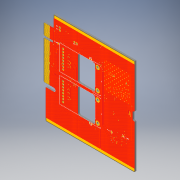
# Autodesk Inventor part: CardStandard
Saved by Autodesk Inventor 2018 (Build 220112000, 112)
## iProperties
Created: 2018-01-15
Part Number: CardStandard
Material: Epoxy Resin
Document SubType Name: Modeling
Designer: Bradley
Density: 1.14 g/cm^3
Appearance: Smooth - Medium Gray
Mass: 15.4834 g
Surface Area: 175.95 cm^2
Volume: 13.582 cm^3
Author: Bradley
Revision Number: 3.1
Autodesk Inventor part; units mm, degrees
ref_plane "YZ Plane" through (0, 0, 0) normal (1, 0, 0) x (0, 1, 0)
ref_plane "XZ Plane" through (0, 0, 0) normal (0, 1, 0) x (-1, 0, 0)
ref_plane "XY Plane" through (0, 0, 0) normal (0, 0, 1) x (1, 0, 0)
sketch "Sketch1" plane through (0, 0, 0) normal (0, 0, 1) x (1, 0, 0)
  line L0 (0, 36.15) -> (10, 36.15)
  line L1 (10, 36.15) -> (10, 47.9)
  line L2 (10, 47.9) -> (90.4, 47.9)
  line L3 (90.4, 47.9) -> (90.4, -47.9)
  line L4 (90.4, -47.9) -> (2, -47.9)
  line L5 (10, -15.15) -> (0, -15.15)
  line L6 (-5.5, 48) -> (90.5, 48) construction
  line L7 (90.5, 48) -> (90.5, -48) construction
  line L8 (90.5, -48) -> (-5.5, -48) construction
  line L9 (-5.5, -48) -> (-5.5, 48) construction
  line L10 (-5.4, 47.9) -> (-3.4, 47.9) construction
  line L11 (-3.4, 47.9) -> (-3.4, -47.9) construction
  line L12 (-3.4, -47.9) -> (-5.4, -47.9) construction
  line L13 (-5.4, -47.9) -> (-5.4, 47.9) construction
  line L14 (-3.4, 38.5) -> (7.85, 38.5) construction
  line L15 (7.85, 38.5) -> (7.85, -17.5) construction
  line L16 (7.85, -17.5) -> (-3.4, -17.5) construction
  line L17 (-3.4, -17.5) -> (-3.4, 38.5) construction
  line L18 (2, -47.9) -> (2, -18.65)
  line L19 (2, -18.65) -> (10, -18.65)
  arc A0 (10, -18.65) -> (10, -15.15) centre (10, -16.9) ccw
  line L20 (0, 24) -> (90.5, 24) construction
  circle A1 centre (-2.5, 47.1) radius 0.9 construction
  circle A2 centre (-0.7, 47.1) radius 0.9 construction
  circle A3 centre (1.1, 47.1) radius 0.9 construction
  circle A4 centre (2.9, 47.1) radius 0.9 construction
  circle A5 centre (4.7, 47.1) radius 0.9 construction
  circle A6 centre (6.5, 47.1) radius 0.9 construction
  circle A7 centre (8.3, 47.1) radius 0.9 construction
  circle A8 centre (-2.5, 45.3) radius 0.9 construction
  circle A9 centre (-0.7, 45.3) radius 0.9 construction
  circle A10 centre (1.1, 45.3) radius 0.9 construction
  circle A11 centre (2.9, 45.3) radius 0.9 construction
  circle A12 centre (4.7, 45.3) radius 0.9 construction
  circle A13 centre (6.5, 45.3) radius 0.9 construction
  circle A14 centre (8.3, 45.3) radius 0.9 construction
  circle A15 centre (-2.5, 43.5) radius 0.9 construction
  circle A16 centre (-0.7, 43.5) radius 0.9 construction
  circle A17 centre (1.1, 43.5) radius 0.9 construction
  circle A18 centre (2.9, 43.5) radius 0.9 construction
  circle A19 centre (4.7, 43.5) radius 0.9 construction
  circle A20 centre (6.5, 43.5) radius 0.9 construction
  circle A21 centre (8.3, 43.5) radius 0.9 construction
  circle A22 centre (-2.5, 41.7) radius 0.9 construction
  circle A23 centre (-0.7, 41.7) radius 0.9 construction
  circle A24 centre (1.1, 41.7) radius 0.9 construction
  circle A25 centre (2.9, 41.7) radius 0.9 construction
  circle A26 centre (4.7, 41.7) radius 0.9 construction
  circle A27 centre (6.5, 41.7) radius 0.9 construction
  circle A28 centre (8.3, 41.7) radius 0.9 construction
  circle A29 centre (-2.5, 39.9) radius 0.9 construction
  circle A30 centre (-0.7, 39.9) radius 0.9 construction
  circle A31 centre (1.1, 39.9) radius 0.9 construction
  circle A32 centre (2.9, 39.9) radius 0.9 construction
  circle A33 centre (4.7, 39.9) radius 0.9 construction
  circle A34 centre (6.5, 39.9) radius 0.9 construction
  circle A35 centre (8.3, 39.9) radius 0.9 construction
  line L21 (0, 36.15) -> (0, 24.95)
  line L22 (0, 24.95) -> (8.4, 24.95)
  arc A36 (8.4, 23.05) -> (8.4, 24.95) centre (8.4, 24) ccw
  line L23 (8.4, 23.05) -> (0, 23.05)
  line L24 (0, 23.05) -> (0, -15.15)
  point P0 (0, 0)
  point P1 (-5.5, 0)
  point P2 (90.4, 0)
  point P3 (90.5, 0)
  dimension "d0" = 51.3
  dimension "d1" = 95.8
  dimension "d3" = 10
  dimension "d20" = 96
  dimension "d21" = 96
  dimension "d22" = 0.1
  dimension "d23" = 0.1
  dimension "d24" = 2
  dimension "d25" = 0.1
  dimension "d28" = 11.25
  dimension "d29" = 56
  dimension "d31" = 9.5
  dimension "d32" = 30.5
  dimension "d34" = 3.5
  dimension "d35" = 12.15
  dimension "d36" = 39.15
  dimension "d37" = 14.5
  dimension "d38" = 1.15
  dimension "d39" = 1.8
  dimension "d42" = 1.8
  dimension "d45" = 1.8
  dimension "d48" = 2
  dimension "d49" = 3.4
  dimension "d50" = 1.9
  dimension "d51" = 8.4
  dimension "d52" = 24
  constraints: 50 end point, 37 centre point, 11 perpendicular, 7 parallel, 6 point on line, 6 tangent, 5 horizontal, 4 point on circle, 3 midpoint, 3 vertical, 2 collinear, 2 horizontal alignment, 68 other
  measures "d0" distance of L5.end L0.start
  measures "d1" distance of L2.end L3.end
  measures "d3" distance of L0.start L0.end
  measures "d20" distance of L6.start L6.end
  measures "d21" distance of L8.end L6.start
  measures "d22" distance between parallel lines of L2 L6
  measures "d23" distance between parallel lines of L7 L3
  measures "d24" distance between parallel lines of L13 L11
  measures "d25" distance between parallel lines of L13 L9
  measures "d28" distance of L15.end L16.end
  measures "d29" distance of L14.end L15.end
  measures "d31" distance between parallel lines of L14 L6
  measures "d32" distance between parallel lines of L8 L16
  measures "d34" distance between parallel lines of L5 L19
  measures "d35" distance between parallel lines of L20 L0
  measures "d36" distance between parallel lines of L5 L20
  measures "d37" distance between parallel lines of L20 L14
  measures "d38" distance between parallel lines of L19 L16
  measures "d39" diameter of A1
  measures "d42" distance of A1.centre A2.centre
  measures "d45" distance of A1.centre A8.centre
  measures "d48" distance between parallel lines of L18 L24
  measures "d49" distance between parallel lines of L24 L11
  measures "d50" distance between parallel lines of L23 L22
  measures "d51" distance of L21.end L22.end
  measures "d52" distance from line of point (0, 0) L20
extrude "Extrusion1" add sketch "Sketch1" along normal mid plane 1.6
chamfer "Chamfer1" distance 0.5 angle 45 4 edges at (0, 36.15, 0) (0, 24.95, 0) (0, 23.05, 0) (0, -15.15, 0)
fillet "Fillet1" radius 0.5 6 edges at (10, 36.15, 0) (10, 47.9, 0) (90.4, 47.9, 0) (90.4, -47.9, 0) (2, -47.9, 0) (2, -18.65, 0)
sketch "Sketch16" plane through (0, 0, 0.8) normal (0, 0, 1) x (1, 0, 0)
  arc A0 (2.5, -18.65) -> (2, -19.15) centre (2.5, -19.15) ccw projected
  line L0 (2, -19.15) -> (2, -47.4) projected
  arc A1 (2, -47.4) -> (2.5, -47.9) centre (2.5, -47.4) ccw projected
  line L1 (2.5, -47.9) -> (89.9, -47.9) projected
  arc A2 (89.9, -47.9) -> (90.4, -47.4) centre (89.9, -47.4) ccw projected
  line L2 (90.4, -47.4) -> (90.4, 47.4) projected
  arc A3 (90.4, 47.4) -> (89.9, 47.9) centre (89.9, 47.4) ccw projected
  line L3 (89.9, 47.9) -> (10.5, 47.9) projected
  arc A4 (10.5, 47.9) -> (10, 47.4) centre (10.5, 47.4) ccw projected
  line L4 (10, 47.4) -> (10, 36.65) projected
  arc A5 (9.5, 36.15) -> (10, 36.65) centre (9.5, 36.65) ccw projected
  line L5 (9.5, 36.15) -> (0.5, 36.15) projected
  line L6 (0, 35.65) -> (0.5, 36.15) projected
  line L7 (0, 35.65) -> (0, 25.45) projected
  line L8 (0.5, 24.95) -> (0, 25.45) projected
  line L9 (0.5, 24.95) -> (8.4, 24.95) projected
  arc A6 (8.4, 23.05) -> (8.4, 24.95) centre (8.4, 24) ccw projected
  line L10 (8.4, 23.05) -> (0.5, 23.05) projected
  line L11 (0, 22.55) -> (0.5, 23.05) projected
  line L12 (0, 22.55) -> (0, -14.65) projected
  line L13 (0.5, -15.15) -> (0, -14.65) projected
  line L14 (0.5, -15.15) -> (10, -15.15) projected
  arc A7 (10, -18.65) -> (10, -15.15) centre (10, -16.9) ccw projected
  line L15 (10, -18.65) -> (2.5, -18.65) projected
  line L16 (36.05, 26.5) -> (49.05, 26.5)
  line L17 (51.05, 24.5) -> (51.05, 3.5)
  line L18 (49.05, 1.5) -> (36.05, 1.5)
  line L19 (34.05, 3.5) -> (34.05, 24.5)
  line L20 (36.05, -1.5) -> (49.05, -1.5)
  line L21 (51.05, -3.5) -> (51.05, -24.5)
  line L22 (49.05, -26.5) -> (36.05, -26.5)
  line L23 (34.05, -24.5) -> (34.05, -3.5)
  line L24 (88.4, 3) -> (88.4, -3)
  arc A8 (88.4, -3) -> (89.4, -4) centre (89.4, -3) ccw
  arc A9 (90.4, -5) -> (89.4, -4) centre (89.4, -5) ccw
  arc A10 (89.4, 4) -> (88.4, 3) centre (89.4, 3) ccw
  line L25 (90.4, -47.4) -> (90.4, 47.4) projected
  arc A11 (89.4, 4) -> (90.4, 5) centre (89.4, 5) ccw
  arc A12 (36.05, 26.5) -> (34.05, 24.5) centre (36.05, 24.5) ccw
  arc A13 (51.05, 24.5) -> (49.05, 26.5) centre (49.05, 24.5) ccw
  arc A14 (49.05, 1.5) -> (51.05, 3.5) centre (49.05, 3.5) ccw
  arc A15 (51.05, -3.5) -> (49.05, -1.5) centre (49.05, -3.5) ccw
  arc A16 (49.05, -26.5) -> (51.05, -24.5) centre (49.05, -24.5) ccw
  arc A17 (34.05, -24.5) -> (36.05, -26.5) centre (36.05, -24.5) ccw
  arc A18 (36.05, -1.5) -> (34.05, -3.5) centre (36.05, -3.5) ccw
  arc A19 (34.05, 3.5) -> (36.05, 1.5) centre (36.05, 3.5) ccw
  point P0 (0, 0)
  point P1 (34.05, -1.5)
  point P2 (51.05, -26.5)
  point P3 (88.4, 0)
  dimension "d145" = 6
  dimension "d146" = 1
  dimension "d147" = 3
  dimension "d148" = 1.5
  dimension "d149" = 34.05
  dimension "d150" = 51.05
  dimension "d151" = 26.5
  dimension "d152" = 2
  constraints: 24 point on circle, 22 tangent, 18 end point, 12 centre point, 10 equal radius, 8 point on line, 4 parallel, 2 horizontal, 2 perpendicular, 1 collinear, 1 horizontal alignment, 1 midpoint, 1 vertical, 1 vertical alignment
  measures "d145" distance of L24.start L24.end
  measures "d146" radius of A11
  measures "d147" distance between parallel lines of L20 L18
  measures "d148" distance from line of point (0, 0) L18
  measures "d149" distance between parallel lines of L19 L12
  measures "d150" distance between parallel lines of L12 L17
  measures "d151" distance from line of point (0, 0) L22
  measures "d152" radius of A12
extrude "Extrusion6" cut sketch "Sketch16" against normal through all contours A9 A8 L24 A10 A11 L2 | L16 A13 L17 A14 L18 A19 L19 A12 | L20 A15 L21 A16 L22 A17 L23 A18
sketch "Sketch19" plane through (0, 0, 0.8) normal (0, 0, 1) x (1, 0, 0)
  line L0 (0, 22.55) -> (0, -14.65) projected
  line L1 (90.4, 5) -> (90.4, 47.4) projected
  line L2 (0, 47.8927) -> (90.4, 47.8927) construction
  line L3 (90.4, 47.8927) -> (90.4, -47.8927) construction
  line L4 (90.4, -47.8927) -> (0, -47.8927) construction
  line L5 (0, -47.8927) -> (0, 47.8927) construction
  point P0 (0, 0)
  constraints: 2 collinear, 1 midpoint, 2 other
decal "Decal4"
sketch "Sketch20" plane through (0, 0, -0.8) normal (0, 0, -1) x (-1, 0, 0)
  line L0 (-90.4, 47.4) -> (-90.4, 5) projected
  line L1 (0, -14.65) -> (0, 22.55) projected
  line L2 (-90.4, 47.8927) -> (0, 47.8927) construction
  line L3 (0, 47.8927) -> (0, -47.8927) construction
  line L4 (0, -47.8927) -> (-90.4, -47.8927) construction
  line L5 (-90.4, -47.8927) -> (-90.4, 47.8927) construction
  point P0 (0, 0)
  constraints: 2 collinear, 1 midpoint, 2 other
decal "Decal5"
sketch "Sketch21" plane through (0, 0, 0.8) normal (0, 0, 1) x (1, 0, 0)
  point P0 (0, 0)
  point P1 (53.55, -24)
  point P2 (53.55, -4)
  point P3 (53.55, 24)
  point P4 (53.55, 4)
  constraints: 4 other
hole "Hole9" at (53.55, -24, 0.8) at (53.55, -4, 0.8) at (53.55, 24, 0.8) at (53.55, 4, 0.8) direction (0, 0, -1) diameter 2.2 end through all
sketch "Sketch22" plane through (0, 0, 0.8) normal (0, 0, 1) x (1, 0, 0)
  point P0 (0, 0)
  point P1 (19.25, -17.81)
  point P2 (32.9, 34.25)
  point P3 (19.25, -12.73)
  point P4 (19.25, -10.19)
  point P5 (19.25, -7.65)
  point P6 (19.25, -5.11)
  point P7 (19.25, -15.27)
  point P8 (19.25, 20.35)
  point P9 (19.25, -20.35)
  point P10 (19.25, -22.89)
  point P11 (19.25, 17.81)
  point P12 (19.25, 15.27)
  point P13 (19.25, 22.89)
  point P14 (19.25, 12.73)
  point P15 (19.25, 10.19)
  point P16 (19.25, 7.65)
  point P17 (19.25, 5.11)
  point P18 (30.5, 34.25)
  point P19 (16, 39.5)
  point P20 (16, 37.05)
  constraints: 20 other
hole "Hole10" at (19.25, -17.81, 0.8) at (32.9, 34.25, 0.8) at (19.25, -12.73, 0.8) at (19.25, -10.19, 0.8) at (19.25, -7.65, 0.8) at (19.25, -5.11, 0.8) at (19.25, -15.27, 0.8) at (19.25, 20.35, 0.8) at (19.25, -20.35, 0.8) at (19.25, -22.89, 0.8) at (19.25, 17.81, 0.8) at (19.25, 15.27, 0.8) at (19.25, 22.89, 0.8) at (19.25, 12.73, 0.8) at (19.25, 10.19, 0.8) at (19.25, 7.65, 0.8) at (19.25, 5.11, 0.8) at (30.5, 34.25, 0.8) at (16, 39.5, 0.8) at (16, 37.05, 0.8) direction (0, 0, -1) diameter 1 end through all
sketch "Sketch23" plane through (0, 0, 0.8) normal (0, 0, 1) x (1, 0, 0)
  point P0 (0, 0)
  point P1 (82, 24.5)
  point P2 (69.5, 24.5)
  constraints: 2 other
hole "Hole11" at (82, 24.5, 0.8) at (69.5, 24.5, 0.8) direction (0, 0, -1) diameter 0.6 end through all
sketch "Sketch24" plane through (0, 0, 0.8) normal (0, 0, 1) x (1, 0, 0)
  point P0 (0, 0)
  point P1 (52.419, -22.869)
  point P2 (51.95, -24)
  point P3 (52.419, -25.131)
  point P4 (55.15, -24)
  point P5 (53.55, -5.6)
  point P6 (54.681, -5.131)
  point P7 (55.15, -4)
  point P8 (54.681, -2.869)
  point P9 (53.55, -2.4)
  point P10 (52.419, -2.869)
  point P11 (54.681, -22.869)
  point P12 (53.55, 22.4)
  point P13 (54.681, 22.869)
  point P14 (55.15, 24)
  point P15 (54.681, 25.131)
  point P16 (53.55, 25.6)
  point P17 (52.419, 25.131)
  point P18 (51.95, -4)
  point P19 (52.419, 22.869)
  point P20 (53.55, 2.4)
  point P21 (54.681, 2.869)
  point P22 (55.15, 4)
  point P23 (54.681, 5.131)
  point P24 (53.55, 5.6)
  point P25 (51.95, 24)
  point P26 (51.95, 4)
  point P27 (52.419, 2.869)
  point P28 (52.419, -5.131)
  point P29 (53.55, -25.6)
  point P30 (54.681, -25.131)
  point P31 (53.55, -22.4)
  point P32 (52.419, 5.131)
  constraints: 32 other
hole "Hole12" at (52.419, -22.869, 0.8) at (51.95, -24, 0.8) at (52.419, -25.131, 0.8) at (55.15, -24, 0.8) at (53.55, -5.6, 0.8) at (54.681, -5.131, 0.8) at (55.15, -4, 0.8) at (54.681, -2.869, 0.8) at (53.55, -2.4, 0.8) at (52.419, -2.869, 0.8) at (54.681, -22.869, 0.8) at (53.55, 22.4, 0.8) at (54.681, 22.869, 0.8) at (55.15, 24, 0.8) at (54.681, 25.131, 0.8) at (53.55, 25.6, 0.8) at (52.419, 25.131, 0.8) at (51.95, -4, 0.8) at (52.419, 22.869, 0.8) at (53.55, 2.4, 0.8) at (54.681, 2.869, 0.8) at (55.15, 4, 0.8) at (54.681, 5.131, 0.8) at (53.55, 5.6, 0.8) at (51.95, 24, 0.8) at (51.95, 4, 0.8) at (52.419, 2.869, 0.8) at (52.419, -5.131, 0.8) at (53.55, -25.6, 0.8) at (54.681, -25.131, 0.8) at (53.55, -22.4, 0.8) at (52.419, 5.131, 0.8) direction (0, 0, -1) diameter 0.35 end through all
sketch "Sketch25" plane through (0, 0, 0.8) normal (0, 0, 1) x (1, 0, 0)
  point P0 (0, 0)
  point P1 (80.65, 14.55)
  point P2 (79.45, 14.55)
  point P3 (79.15, 12.8)
  point P4 (79.1, 11.55)
  point P5 (77.3, 14.15)
  point P6 (76.1, 14.15)
  point P7 (77.25, 12.15)
  point P8 (77.25, 10.95)
  point P9 (74.55, 13)
  point P10 (72.7, 14.55)
  point P11 (69.6, 14.35)
  point P12 (69.8, 13)
  point P13 (69.8, 11.1)
  point P14 (72.3, 11.4)
  point P15 (66.9, 23.8)
  point P16 (68.5, 23.8)
  point P17 (64.9, 24.9)
  point P18 (68.5, 25.1)
  point P19 (66.9, 25.1)
  point P20 (64.9, 23.6)
  point P21 (82.7, 23.6)
  point P22 (81.3, 23.6)
  point P23 (82, 25.6)
  point P24 (82.7, 19.4)
  point P25 (81.3, 18.8)
  point P26 (83.8, 16.4)
  point P27 (85, 17)
  point P28 (85.05, 14.2)
  point P29 (81.1, 16.2)
  point P30 (77.95, 16.35)
  point P31 (75.05, 16.35)
  point P32 (71.85, 15.55)
  point P33 (66.5, 13.7)
  point P34 (65.6, 12.3)
  point P35 (70.6, 24.5)
  point P36 (84.5, 32)
  point P37 (76.5, 32)
  point P38 (68.5, 32)
  point P39 (72.5, 32)
  point P40 (80.5, 32)
  point P41 (64.5, 32)
  point P42 (82.5, 30)
  point P43 (74.5, 30)
  point P44 (66.5, 30)
  point P45 (70.5, 30)
  point P46 (78.5, 30)
  point P47 (62.5, 30)
  point P48 (84.5, 28)
  point P49 (76.5, 28)
  point P50 (68.5, 28)
  point P51 (72.5, 28)
  point P52 (80.5, 28)
  point P53 (64.5, 28)
  point P54 (74.5, 26)
  point P55 (66.5, 26)
  point P56 (70.5, 26)
  point P57 (78.5, 26)
  point P58 (62.5, 26)
  point P59 (84.5, 24)
  point P60 (76.5, 24)
  point P61 (72.5, 24)
  point P62 (74.5, 22)
  point P63 (66.5, 22)
  point P64 (70.5, 22)
  point P65 (78.5, 22)
  point P66 (62.5, 22)
  point P67 (84.5, 20)
  point P68 (76.5, 20)
  point P69 (68.5, 20)
  point P70 (72.5, 20)
  point P71 (80.5, 20)
  point P72 (64.5, 20)
  point P73 (74.5, 18)
  point P74 (66.5, 18)
  point P75 (70.5, 18)
  point P76 (78.5, 18)
  point P77 (62.5, 18)
  point P78 (84.5, 8)
  point P79 (76.5, 8)
  point P80 (68.5, 8)
  point P81 (72.5, 8)
  point P82 (80.5, 8)
  point P83 (64.5, 8)
  point P84 (82.5, 10)
  point P85 (74.5, 10)
  point P86 (66.5, 10)
  point P87 (70.5, 10)
  point P88 (78.5, 10)
  point P89 (62.5, 10)
  point P90 (82.5, 34)
  point P91 (74.5, 34)
  point P92 (66.5, 34)
  point P93 (70.5, 34)
  point P94 (56.2, 27.1)
  point P95 (62.5, 34)
  point P96 (60.5, 32)
  point P97 (60.5, 28)
  point P98 (60.5, 24)
  point P99 (60.5, 20)
  point P100 (60.5, 16)
  point P101 (62.5, 14)
  point P102 (60.5, 12)
  point P103 (64.5, 12)
  point P104 (64.5, 16)
  point P105 (13.5, 24.2)
  point P106 (15.3, 2.5)
  point P107 (15.3, -4.8)
  point P108 (55.3, -27)
  point P109 (73.075, -22.125)
  point P110 (77.7, -26.1)
  point P111 (25, 9.9)
  point P112 (25, 12.8)
  point P113 (25, 15.9)
  point P114 (24.59, 18.9)
  point P115 (24.6, -9.1)
  point P116 (25, -18.1)
  point P117 (25, -15.1)
  point P118 (25, -12.1)
  point P119 (80.4, -20.2)
  point P120 (80.4, -17.9)
  point P121 (62.6, 1.8)
  point P122 (60.2, 3.5)
  point P123 (25.25, 1.4)
  point P124 (25.25, -1.4)
  point P125 (28.5, 1.4)
  point P126 (13.8, 20)
  point P127 (67.5, -26.2)
  point P128 (58.86, 23)
  point P129 (67, -31)
  point P130 (72.9, -30.3)
  point P131 (69.3, -28.5)
  point P132 (67, -28.5)
  point P133 (55.5, 29.3)
  point P134 (57.7, 27.5)
  point P135 (57.7, 25.6)
  point P136 (72.5, -32.1)
  point P137 (87.6, 7.7)
  point P138 (70.3, -30.7)
  point P139 (68.7, -33.25)
  point P140 (70.432, -27.94)
  point P141 (77.1, -30.9)
  point P142 (72.3, -26.4)
  point P143 (58.3, 24.9)
  point P144 (67, -32.3)
  point P145 (72.4, -30.9)
  point P146 (69.3, -29.8)
  point P147 (51.75, -29.75)
  point P148 (70.001, -7.599)
  point P149 (69.209, -8.391)
  point P150 (77.45, -23.85)
  point P151 (6, -2.5)
  point P152 (30.5, -2.4)
  point P153 (26.4, 14.45)
  point P154 (6, -3.5)
  point P155 (31.1, -3)
  point P156 (29.9, -3)
  point P157 (29.9, -1.8)
  point P158 (26.4, 13.6)
  point P159 (6, -4.5)
  point P160 (31.7, -3.6)
  point P161 (29.3, -3.6)
  point P162 (29.3, -1.2)
  point P163 (26.4, 11.45)
  point P164 (58, 30.4)
  point P165 (17.6, 8.9)
  point P166 (26.4, 10.1)
  point P167 (9.8, 5.2)
  point P168 (20.7, -1.4)
  point P169 (24.5, -5.2)
  point P170 (6, 34.5)
  point P171 (6, 4.5)
  point P172 (6, 3.5)
  point P173 (27.596, 0.396)
  point P174 (26.804, -0.396)
  point P175 (25.3, 18.4)
  point P176 (25.8, 15.4)
  point P177 (25.8, 12.4)
  point P178 (25.3, -9.6)
  point P179 (25.8, -12.6)
  point P180 (25.8, -15.6)
  point P181 (6, 35.5)
  point P182 (25.2, 21)
  point P183 (26.4, -5.9)
  point P184 (32.4, -0.76)
  point P185 (70.6, 4.6)
  point P186 (70.75, 6.25)
  point P187 (6, 33.5)
  point P188 (6, 32.5)
  point P189 (6, 31.5)
  point P190 (6, 30.5)
  point P191 (6, 29.5)
  point P192 (6, 28.5)
  point P193 (6, 27.5)
  point P194 (6, 26.5)
  point P195 (6, 20.5)
  point P196 (6, 19.5)
  point P197 (6, 18.5)
  point P198 (6, 17.5)
  point P199 (6, 16.5)
  constraints: 244 other
hole "Hole13" at (80.65, 14.55, 0.8) at (79.45, 14.55, 0.8) at (79.15, 12.8, 0.8) at (79.1, 11.55, 0.8) at (77.3, 14.15, 0.8) at (76.1, 14.15, 0.8) at (77.25, 12.15, 0.8) at (77.25, 10.95, 0.8) at (74.55, 13, 0.8) at (72.7, 14.55, 0.8) at (69.6, 14.35, 0.8) at (69.8, 13, 0.8) at (69.8, 11.1, 0.8) at (72.3, 11.4, 0.8) at (66.9, 23.8, 0.8) at (68.5, 23.8, 0.8) at (64.9, 24.9, 0.8) at (68.5, 25.1, 0.8) at (66.9, 25.1, 0.8) at (64.9, 23.6, 0.8) at (82.7, 23.6, 0.8) at (81.3, 23.6, 0.8) at (82, 25.6, 0.8) at (82.7, 19.4, 0.8) at (81.3, 18.8, 0.8) at (83.8, 16.4, 0.8) at (85, 17, 0.8) at (85.05, 14.2, 0.8) at (81.1, 16.2, 0.8) at (77.95, 16.35, 0.8) at (75.05, 16.35, 0.8) at (71.85, 15.55, 0.8) at (66.5, 13.7, 0.8) at (65.6, 12.3, 0.8) at (70.6, 24.5, 0.8) at (84.5, 32, 0.8) at (76.5, 32, 0.8) at (68.5, 32, 0.8) at (72.5, 32, 0.8) at (80.5, 32, 0.8) at (64.5, 32, 0.8) at (82.5, 30, 0.8) at (74.5, 30, 0.8) at (66.5, 30, 0.8) at (70.5, 30, 0.8) at (78.5, 30, 0.8) at (62.5, 30, 0.8) at (84.5, 28, 0.8) at (76.5, 28, 0.8) at (68.5, 28, 0.8) direction (0, 0, -1) diameter 0.3 end through all and at (72.5, 28, 0.8) (80.5, 28, 0.8) (64.5, 28, 0.8) (74.5, 26, 0.8) (66.5, 26, 0.8) (70.5, 26, 0.8) (78.5, 26, 0.8) (62.5, 26, 0.8) (84.5, 24, 0.8) (76.5, 24, 0.8) (72.5, 24, 0.8) (74.5, 22, 0.8) (66.5, 22, 0.8) (70.5, 22, 0.8) (78.5, 22, 0.8) (62.5, 22, 0.8) (84.5, 20, 0.8) (76.5, 20, 0.8) (68.5, 20, 0.8) (72.5, 20, 0.8) (80.5, 20, 0.8) (64.5, 20, 0.8) (74.5, 18, 0.8) (66.5, 18, 0.8) (70.5, 18, 0.8) (78.5, 18, 0.8) (62.5, 18, 0.8) (84.5, 8, 0.8) (76.5, 8, 0.8) (68.5, 8, 0.8) (72.5, 8, 0.8) (80.5, 8, 0.8) (64.5, 8, 0.8) (82.5, 10, 0.8) (74.5, 10, 0.8) (66.5, 10, 0.8) (70.5, 10, 0.8) (78.5, 10, 0.8) (62.5, 10, 0.8) (82.5, 34, 0.8) (74.5, 34, 0.8) (66.5, 34, 0.8) (70.5, 34, 0.8) (56.2, 27.1, 0.8) (62.5, 34, 0.8) (60.5, 32, 0.8) (60.5, 28, 0.8) (60.5, 24, 0.8) (60.5, 20, 0.8) (60.5, 16, 0.8) (62.5, 14, 0.8) (60.5, 12, 0.8) (64.5, 12, 0.8) (64.5, 16, 0.8) (13.5, 24.2, 0.8) (15.3, 2.5, 0.8) (15.3, -4.8, 0.8) (55.3, -27, 0.8) (73.075, -22.125, 0.8) (77.7, -26.1, 0.8) (25, 9.9, 0.8) (25, 12.8, 0.8) (25, 15.9, 0.8) (24.59, 18.9, 0.8) (24.6, -9.1, 0.8) (25, -18.1, 0.8) (25, -15.1, 0.8) (25, -12.1, 0.8) (80.4, -20.2, 0.8) (80.4, -17.9, 0.8) (62.6, 1.8, 0.8) (60.2, 3.5, 0.8) (25.25, 1.4, 0.8) (25.25, -1.4, 0.8) (28.5, 1.4, 0.8) (13.8, 20, 0.8) (67.5, -26.2, 0.8) (58.86, 23, 0.8) (67, -31, 0.8) (72.9, -30.3, 0.8) (69.3, -28.5, 0.8) (67, -28.5, 0.8) (55.5, 29.3, 0.8) (57.7, 27.5, 0.8) (57.7, 25.6, 0.8) (72.5, -32.1, 0.8) (87.6, 7.7, 0.8) (70.3, -30.7, 0.8) (68.7, -33.25, 0.8) (70.432, -27.94, 0.8) (77.1, -30.9, 0.8) (72.3, -26.4, 0.8) (58.3, 24.9, 0.8) (67, -32.3, 0.8) (72.4, -30.9, 0.8) (69.3, -29.8, 0.8) (51.75, -29.75, 0.8) (70.001, -7.599, 0.8) (69.209, -8.391, 0.8) (77.45, -23.85, 0.8) (6, -2.5, 0.8) (30.5, -2.4, 0.8) (26.4, 14.45, 0.8) (6, -3.5, 0.8) (31.1, -3, 0.8) (29.9, -3, 0.8) (29.9, -1.8, 0.8) (26.4, 13.6, 0.8) (6, -4.5, 0.8) (31.7, -3.6, 0.8) (29.3, -3.6, 0.8) (29.3, -1.2, 0.8) (26.4, 11.45, 0.8) (58, 30.4, 0.8) (17.6, 8.9, 0.8) (26.4, 10.1, 0.8) (9.8, 5.2, 0.8) (20.7, -1.4, 0.8) (24.5, -5.2, 0.8) (6, 34.5, 0.8) (6, 4.5, 0.8) (6, 3.5, 0.8) (27.596, 0.396, 0.8) (26.804, -0.396, 0.8) (25.3, 18.4, 0.8) (25.8, 15.4, 0.8) (25.8, 12.4, 0.8) (25.3, -9.6, 0.8) (25.8, -12.6, 0.8) (25.8, -15.6, 0.8) (6, 35.5, 0.8) (25.2, 21, 0.8) (26.4, -5.9, 0.8) (32.4, -0.76, 0.8) (70.6, 4.6, 0.8) (70.75, 6.25, 0.8) (6, 33.5, 0.8) (6, 32.5, 0.8) (6, 31.5, 0.8) (6, 30.5, 0.8) (6, 29.5, 0.8) (6, 28.5, 0.8) (6, 27.5, 0.8) (6, 26.5, 0.8) (6, 20.5, 0.8) (6, 19.5, 0.8) (6, 18.5, 0.8) (6, 17.5, 0.8) (6, 16.5, 0.8) (6, 15.5, 0.8) (6, 14.5, 0.8) (60.7, 1.2, 0.8) (60.7, -1.2, 0.8) (6, 25.55, 0.8) (77.9, -27.6, 0.8) (82, -26.8, 0.8) (78.5, 34, 0.8) (74.4, -11, 0.8) (69.1, -6, 0.8) (17, 27.19, 0.8) (10.6, 25.9, 0.8) (6, 22.45, 0.8) (24.05, 9.7, 0.8) (24.05, 12.7, 0.8) (24.05, 15.7, 0.8) (24.05, 18.35, 0.8) (6, 21.5, 0.8) (24.05, -18.3, 0.8) (24.05, -15.3, 0.8) (24.05, -12.3, 0.8) (24.05, -9.65, 0.8) (8.8, 2.3, 0.8) (56.2, -44.3, 0.8) (56.6, 42.9, 0.8) (57.7, 44.4, 0.8) (24.2, 38.74, 0.8) (22, 39.4, 0.8) (6.2, 13.5, 0.8) (6.2, 12.5, 0.8) (6.2, 11.5, 0.8) (9.95, 22.05, 0.8) (12.35, 15.75, 0.8) (7.7, 2.3, 0.8) (10.8, 34.1, 0.8) (56.8, 28.2, 0.8) (19.95, 27.75, 0.8) (35.3, 28.2, 0.8) (48.3, -27.75, 0.8) (80, -24, 0.8) (82.6, -24, 0.8) (82.9, 14.75, 0.8) (81.05, 11.5, 0.8) (82.9, 13.25, 0.8) (26.4, -16.9, 0.8)
sketch "Sketch26" plane through (0, 0, 0) normal (0, 0, 1) x (1, 0, 0)
  circle A0 centre (82.9, 13.25) radius 0.15 projected
  circle A1 centre (82.9, 14.75) radius 0.15 projected
  circle A2 centre (80, -24) radius 0.15 projected
  circle A3 centre (35.3, 28.2) radius 0.15 projected
  circle A4 centre (56.8, 28.2) radius 0.15 projected
  circle A5 centre (7.7, 2.3) radius 0.15 projected
  circle A6 centre (9.95, 22.05) radius 0.15 projected
  circle A7 centre (6.2, 12.5) radius 0.15 projected
  circle A8 centre (22, 39.4) radius 0.15 projected
  circle A9 centre (57.7, 44.4) radius 0.15 projected
  circle A10 centre (56.2, -44.3) radius 0.15 projected
  circle A11 centre (24.05, -9.65) radius 0.15 projected
  circle A12 centre (24.05, -15.3) radius 0.15 projected
  circle A13 centre (6, 21.5) radius 0.15 projected
  circle A14 centre (24.05, 15.7) radius 0.15 projected
  circle A15 centre (24.05, 9.7) radius 0.15 projected
  circle A16 centre (10.6, 25.9) radius 0.15 projected
  circle A17 centre (69.1, -6) radius 0.15 projected
  circle A18 centre (78.5, 34) radius 0.15 projected
  circle A19 centre (77.9, -27.6) radius 0.15 projected
  circle A20 centre (60.7, -1.2) radius 0.15 projected
  circle A21 centre (6, 14.5) radius 0.15 projected
  circle A22 centre (6, 16.5) radius 0.15 projected
  circle A23 centre (6, 18.5) radius 0.15 projected
  circle A24 centre (6, 20.5) radius 0.15 projected
  circle A25 centre (6, 27.5) radius 0.15 projected
  circle A26 centre (6, 29.5) radius 0.15 projected
  circle A27 centre (6, 31.5) radius 0.15 projected
  circle A28 centre (6, 33.5) radius 0.15 projected
  circle A29 centre (70.6, 4.6) radius 0.15 projected
  circle A30 centre (26.4, -5.9) radius 0.15 projected
  circle A31 centre (6, 35.5) radius 0.15 projected
  circle A32 centre (25.8, -12.6) radius 0.15 projected
  circle A33 centre (25.8, 12.4) radius 0.15 projected
  circle A34 centre (25.3, 18.4) radius 0.15 projected
  circle A35 centre (27.596, 0.396) radius 0.15 projected
  circle A36 centre (6, 4.5) radius 0.15 projected
  circle A37 centre (24.5, -5.2) radius 0.15 projected
  circle A38 centre (9.8, 5.2) radius 0.15 projected
  circle A39 centre (17.6, 8.9) radius 0.15 projected
  circle A40 centre (26.4, 11.45) radius 0.15 projected
  circle A41 centre (29.3, -3.6) radius 0.15 projected
  circle A42 centre (6, -4.5) radius 0.15 projected
  circle A43 centre (29.9, -1.8) radius 0.15 projected
  circle A44 centre (31.1, -3) radius 0.15 projected
  circle A45 centre (26.4, 14.45) radius 0.15 projected
  circle A46 centre (6, -2.5) radius 0.15 projected
  circle A47 centre (69.209, -8.391) radius 0.15 projected
  circle A48 centre (51.75, -29.75) radius 0.15 projected
  circle A49 centre (72.4, -30.9) radius 0.15 projected
  circle A50 centre (58.3, 24.9) radius 0.15 projected
  circle A51 centre (77.1, -30.9) radius 0.15 projected
  circle A52 centre (68.7, -33.25) radius 0.15 projected
  circle A53 centre (87.6, 7.7) radius 0.15 projected
  circle A54 centre (57.7, 25.6) radius 0.15 projected
  circle A55 centre (55.5, 29.3) radius 0.15 projected
  circle A56 centre (69.3, -28.5) radius 0.15 projected
  circle A57 centre (67, -31) radius 0.15 projected
  circle A58 centre (67.5, -26.2) radius 0.15 projected
  circle A59 centre (28.5, 1.4) radius 0.15 projected
  circle A60 centre (25.25, 1.4) radius 0.15 projected
  circle A61 centre (62.6, 1.8) radius 0.15 projected
  circle A62 centre (80.4, -20.2) radius 0.15 projected
  circle A63 centre (25, -15.1) radius 0.15 projected
  circle A64 centre (24.6, -9.1) radius 0.15 projected
  circle A65 centre (25, 15.9) radius 0.15 projected
  circle A66 centre (25, 9.9) radius 0.15 projected
  circle A67 centre (73.075, -22.125) radius 0.15 projected
  circle A68 centre (15.3, -4.8) radius 0.15 projected
  circle A69 centre (13.5, 24.2) radius 0.15 projected
  circle A70 centre (64.5, 12) radius 0.15 projected
  circle A71 centre (62.5, 14) radius 0.15 projected
  circle A72 centre (60.5, 20) radius 0.15 projected
  circle A73 centre (60.5, 28) radius 0.15 projected
  circle A74 centre (62.5, 34) radius 0.15 projected
  circle A75 centre (70.5, 34) radius 0.15 projected
  circle A76 centre (74.5, 34) radius 0.15 projected
  circle A77 centre (62.5, 10) radius 0.15 projected
  circle A78 centre (70.5, 10) radius 0.15 projected
  circle A79 centre (74.5, 10) radius 0.15 projected
  circle A80 centre (64.5, 8) radius 0.15 projected
  circle A81 centre (72.5, 8) radius 0.15 projected
  circle A82 centre (76.5, 8) radius 0.15 projected
  circle A83 centre (62.5, 18) radius 0.15 projected
  circle A84 centre (70.5, 18) radius 0.15 projected
  circle A85 centre (74.5, 18) radius 0.15 projected
  circle A86 centre (80.5, 20) radius 0.15 projected
  circle A87 centre (68.5, 20) radius 0.15 projected
  circle A88 centre (84.5, 20) radius 0.15 projected
  circle A89 centre (78.5, 22) radius 0.15 projected
  circle A90 centre (66.5, 22) radius 0.15 projected
  circle A91 centre (72.5, 24) radius 0.15 projected
  circle A92 centre (84.5, 24) radius 0.15 projected
  circle A93 centre (78.5, 26) radius 0.15 projected
  circle A94 centre (66.5, 26) radius 0.15 projected
  circle A95 centre (64.5, 28) radius 0.15 projected
  circle A96 centre (72.5, 28) radius 0.15 projected
  circle A97 centre (76.5, 28) radius 0.15 projected
  circle A98 centre (62.5, 30) radius 0.15 projected
  circle A99 centre (70.5, 30) radius 0.15 projected
  circle A100 centre (74.5, 30) radius 0.15 projected
  circle A101 centre (64.5, 32) radius 0.15 projected
  circle A102 centre (72.5, 32) radius 0.15 projected
  circle A103 centre (76.5, 32) radius 0.15 projected
  circle A104 centre (70.6, 24.5) radius 0.15 projected
  circle A105 centre (66.5, 13.7) radius 0.15 projected
  circle A106 centre (75.05, 16.35) radius 0.15 projected
  circle A107 centre (81.1, 16.2) radius 0.15 projected
  circle A108 centre (85, 17) radius 0.15 projected
  circle A109 centre (81.3, 18.8) radius 0.15 projected
  circle A110 centre (82, 25.6) radius 0.15 projected
  circle A111 centre (82.7, 23.6) radius 0.15 projected
  circle A112 centre (66.9, 25.1) radius 0.15 projected
  circle A113 centre (64.9, 24.9) radius 0.15 projected
  circle A114 centre (66.9, 23.8) radius 0.15 projected
  circle A115 centre (69.8, 11.1) radius 0.15 projected
  circle A116 centre (69.6, 14.35) radius 0.15 projected
  circle A117 centre (74.55, 13) radius 0.15 projected
  circle A118 centre (77.25, 12.15) radius 0.15 projected
  circle A119 centre (77.3, 14.15) radius 0.15 projected
  circle A120 centre (79.15, 12.8) radius 0.15 projected
  circle A121 centre (80.65, 14.55) radius 0.15 projected
  circle A122 centre (79.45, 14.55) radius 0.15 projected
  circle A123 centre (79.1, 11.55) radius 0.15 projected
  circle A124 centre (76.1, 14.15) radius 0.15 projected
  circle A125 centre (77.25, 10.95) radius 0.15 projected
  circle A126 centre (72.7, 14.55) radius 0.15 projected
  circle A127 centre (69.8, 13) radius 0.15 projected
  circle A128 centre (72.3, 11.4) radius 0.15 projected
  circle A129 centre (68.5, 23.8) radius 0.15 projected
  circle A130 centre (68.5, 25.1) radius 0.15 projected
  circle A131 centre (64.9, 23.6) radius 0.15 projected
  circle A132 centre (81.3, 23.6) radius 0.15 projected
  circle A133 centre (82.7, 19.4) radius 0.15 projected
  circle A134 centre (83.8, 16.4) radius 0.15 projected
  circle A135 centre (85.05, 14.2) radius 0.15 projected
  circle A136 centre (77.95, 16.35) radius 0.15 projected
  circle A137 centre (71.85, 15.55) radius 0.15 projected
  circle A138 centre (65.6, 12.3) radius 0.15 projected
  circle A139 centre (84.5, 32) radius 0.15 projected
  circle A140 centre (68.5, 32) radius 0.15 projected
  circle A141 centre (80.5, 32) radius 0.15 projected
  circle A142 centre (82.5, 30) radius 0.15 projected
  circle A143 centre (66.5, 30) radius 0.15 projected
  circle A144 centre (78.5, 30) radius 0.15 projected
  circle A145 centre (84.5, 28) radius 0.15 projected
  circle A146 centre (68.5, 28) radius 0.15 projected
  circle A147 centre (80.5, 28) radius 0.15 projected
  circle A148 centre (74.5, 26) radius 0.15 projected
  circle A149 centre (70.5, 26) radius 0.15 projected
  circle A150 centre (62.5, 26) radius 0.15 projected
  circle A151 centre (76.5, 24) radius 0.15 projected
  circle A152 centre (74.5, 22) radius 0.15 projected
  circle A153 centre (70.5, 22) radius 0.15 projected
  circle A154 centre (62.5, 22) radius 0.15 projected
  circle A155 centre (76.5, 20) radius 0.15 projected
  circle A156 centre (72.5, 20) radius 0.15 projected
  circle A157 centre (64.5, 20) radius 0.15 projected
  circle A158 centre (66.5, 18) radius 0.15 projected
  circle A159 centre (78.5, 18) radius 0.15 projected
  circle A160 centre (84.5, 8) radius 0.15 projected
  circle A161 centre (68.5, 8) radius 0.15 projected
  circle A162 centre (80.5, 8) radius 0.15 projected
  circle A163 centre (82.5, 10) radius 0.15 projected
  circle A164 centre (66.5, 10) radius 0.15 projected
  circle A165 centre (78.5, 10) radius 0.15 projected
  circle A166 centre (82.5, 34) radius 0.15 projected
  circle A167 centre (66.5, 34) radius 0.15 projected
  circle A168 centre (56.2, 27.1) radius 0.15 projected
  circle A169 centre (60.5, 32) radius 0.15 projected
  circle A170 centre (60.5, 24) radius 0.15 projected
  circle A171 centre (60.5, 16) radius 0.15 projected
  circle A172 centre (60.5, 12) radius 0.15 projected
  circle A173 centre (64.5, 16) radius 0.15 projected
  circle A174 centre (15.3, 2.5) radius 0.15 projected
  circle A175 centre (55.3, -27) radius 0.15 projected
  circle A176 centre (77.7, -26.1) radius 0.15 projected
  circle A177 centre (25, 12.8) radius 0.15 projected
  circle A178 centre (24.59, 18.9) radius 0.15 projected
  circle A179 centre (25, -18.1) radius 0.15 projected
  circle A180 centre (25, -12.1) radius 0.15 projected
  circle A181 centre (80.4, -17.9) radius 0.15 projected
  circle A182 centre (60.2, 3.5) radius 0.15 projected
  circle A183 centre (25.25, -1.4) radius 0.15 projected
  circle A184 centre (13.8, 20) radius 0.15 projected
  circle A185 centre (58.86, 23) radius 0.15 projected
  circle A186 centre (72.9, -30.3) radius 0.15 projected
  circle A187 centre (67, -28.5) radius 0.15 projected
  circle A188 centre (57.7, 27.5) radius 0.15 projected
  circle A189 centre (72.5, -32.1) radius 0.15 projected
  circle A190 centre (70.3, -30.7) radius 0.15 projected
  circle A191 centre (70.432, -27.94) radius 0.15 projected
  circle A192 centre (72.3, -26.4) radius 0.15 projected
  circle A193 centre (67, -32.3) radius 0.15 projected
  circle A194 centre (69.3, -29.8) radius 0.15 projected
  circle A195 centre (70.001, -7.599) radius 0.15 projected
  circle A196 centre (77.45, -23.85) radius 0.15 projected
  circle A197 centre (30.5, -2.4) radius 0.15 projected
  circle A198 centre (6, -3.5) radius 0.15 projected
  circle A199 centre (29.9, -3) radius 0.15 projected
  circle A200 centre (26.4, 13.6) radius 0.15 projected
  circle A201 centre (31.7, -3.6) radius 0.15 projected
  circle A202 centre (29.3, -1.2) radius 0.15 projected
  circle A203 centre (58, 30.4) radius 0.15 projected
  circle A204 centre (26.4, 10.1) radius 0.15 projected
  circle A205 centre (20.7, -1.4) radius 0.15 projected
  circle A206 centre (6, 34.5) radius 0.15 projected
  circle A207 centre (6, 3.5) radius 0.15 projected
  circle A208 centre (26.804, -0.396) radius 0.15 projected
  circle A209 centre (25.8, 15.4) radius 0.15 projected
  circle A210 centre (25.3, -9.6) radius 0.15 projected
  circle A211 centre (25.8, -15.6) radius 0.15 projected
  circle A212 centre (25.2, 21) radius 0.15 projected
  circle A213 centre (32.4, -0.76) radius 0.15 projected
  circle A214 centre (70.75, 6.25) radius 0.15 projected
  circle A215 centre (6, 32.5) radius 0.15 projected
  circle A216 centre (6, 30.5) radius 0.15 projected
  circle A217 centre (6, 28.5) radius 0.15 projected
  circle A218 centre (6, 26.5) radius 0.15 projected
  circle A219 centre (6, 19.5) radius 0.15 projected
  circle A220 centre (6, 17.5) radius 0.15 projected
  circle A221 centre (6, 15.5) radius 0.15 projected
  circle A222 centre (60.7, 1.2) radius 0.15 projected
  circle A223 centre (6, 25.55) radius 0.15 projected
  circle A224 centre (82, -26.8) radius 0.15 projected
  circle A225 centre (74.4, -11) radius 0.15 projected
  circle A226 centre (17, 27.19) radius 0.15 projected
  circle A227 centre (6, 22.45) radius 0.15 projected
  circle A228 centre (24.05, 12.7) radius 0.15 projected
  circle A229 centre (24.05, 18.35) radius 0.15 projected
  circle A230 centre (24.05, -18.3) radius 0.15 projected
  circle A231 centre (24.05, -12.3) radius 0.15 projected
  circle A232 centre (8.8, 2.3) radius 0.15 projected
  circle A233 centre (56.6, 42.9) radius 0.15 projected
  circle A234 centre (24.2, 38.74) radius 0.15 projected
  circle A235 centre (6.2, 13.5) radius 0.15 projected
  circle A236 centre (6.2, 11.5) radius 0.15 projected
  circle A237 centre (12.35, 15.75) radius 0.15 projected
  circle A238 centre (10.8, 34.1) radius 0.15 projected
  circle A239 centre (19.95, 27.75) radius 0.15 projected
  circle A240 centre (48.3, -27.75) radius 0.15 projected
  circle A241 centre (82.6, -24) radius 0.15 projected
  circle A242 centre (81.05, 11.5) radius 0.15 projected
  circle A243 centre (26.4, -16.9) radius 0.15 projected
  circle A244 centre (53.55, -22.4) radius 0.175 projected
  circle A245 centre (53.55, -25.6) radius 0.175 projected
  circle A246 centre (52.419, 2.869) radius 0.175 projected
  circle A247 centre (51.95, 24) radius 0.175 projected
  circle A248 centre (54.681, 5.131) radius 0.175 projected
  circle A249 centre (54.681, 2.869) radius 0.175 projected
  circle A250 centre (52.419, 22.869) radius 0.175 projected
  circle A251 centre (52.419, 25.131) radius 0.175 projected
  circle A252 centre (54.681, 25.131) radius 0.175 projected
  circle A253 centre (54.681, 22.869) radius 0.175 projected
  circle A254 centre (54.681, -22.869) radius 0.175 projected
  circle A255 centre (53.55, -2.4) radius 0.175 projected
  circle A256 centre (55.15, -4) radius 0.175 projected
  circle A257 centre (53.55, -5.6) radius 0.175 projected
  circle A258 centre (52.419, -25.131) radius 0.175 projected
  circle A259 centre (52.419, -22.869) radius 0.175 projected
  circle A260 centre (51.95, -24) radius 0.175 projected
  circle A261 centre (55.15, -24) radius 0.175 projected
  circle A262 centre (54.681, -5.131) radius 0.175 projected
  circle A263 centre (54.681, -2.869) radius 0.175 projected
  circle A264 centre (52.419, -2.869) radius 0.175 projected
  circle A265 centre (53.55, 22.4) radius 0.175 projected
  circle A266 centre (55.15, 24) radius 0.175 projected
  circle A267 centre (53.55, 25.6) radius 0.175 projected
  circle A268 centre (51.95, -4) radius 0.175 projected
  circle A269 centre (53.55, 2.4) radius 0.175 projected
  circle A270 centre (55.15, 4) radius 0.175 projected
  circle A271 centre (53.55, 5.6) radius 0.175 projected
  circle A272 centre (51.95, 4) radius 0.175 projected
  circle A273 centre (52.419, -5.131) radius 0.175 projected
  circle A274 centre (54.681, -25.131) radius 0.175 projected
  circle A275 centre (52.419, 5.131) radius 0.175 projected
  circle A276 centre (82, 24.5) radius 0.3 projected
  circle A277 centre (69.5, 24.5) radius 0.3 projected
  circle A278 centre (16, 39.5) radius 0.5 projected
  circle A279 centre (19.25, 5.11) radius 0.5 projected
  circle A280 centre (19.25, 10.19) radius 0.5 projected
  circle A281 centre (19.25, 22.89) radius 0.5 projected
  circle A282 centre (19.25, 17.81) radius 0.5 projected
  circle A283 centre (19.25, -20.35) radius 0.5 projected
  circle A284 centre (19.25, -15.27) radius 0.5 projected
  circle A285 centre (19.25, -7.65) radius 0.5 projected
  circle A286 centre (19.25, -12.73) radius 0.5 projected
  circle A287 centre (19.25, -17.81) radius 0.5 projected
  circle A288 centre (32.9, 34.25) radius 0.5 projected
  circle A289 centre (19.25, -10.19) radius 0.5 projected
  circle A290 centre (19.25, -5.11) radius 0.5 projected
  circle A291 centre (19.25, 20.35) radius 0.5 projected
  circle A292 centre (19.25, -22.89) radius 0.5 projected
  circle A293 centre (19.25, 15.27) radius 0.5 projected
  circle A294 centre (19.25, 12.73) radius 0.5 projected
  circle A295 centre (19.25, 7.65) radius 0.5 projected
  circle A296 centre (30.5, 34.25) radius 0.5 projected
  circle A297 centre (16, 37.05) radius 0.5 projected
  circle A298 centre (53.55, 24) radius 1.1 projected
  circle A299 centre (53.55, -24) radius 1.1 projected
  circle A300 centre (53.55, -4) radius 1.1 projected
  circle A301 centre (53.55, 4) radius 1.1 projected
  arc A302 (90.4, -5) -> (89.4, -4) centre (89.4, -5) ccw projected
  arc A303 (88.4, -3) -> (89.4, -4) centre (89.4, -3) ccw projected
  line L0 (88.4, -3) -> (88.4, 3) projected
  arc A304 (89.4, 4) -> (88.4, 3) centre (89.4, 3) ccw projected
  arc A305 (89.4, 4) -> (90.4, 5) centre (89.4, 5) ccw projected
  line L1 (90.4, 5) -> (90.4, 47.4) projected
  arc A306 (90.4, 47.4) -> (89.9, 47.9) centre (89.9, 47.4) ccw projected
  line L2 (89.9, 47.9) -> (10.5, 47.9) projected
  arc A307 (10.5, 47.9) -> (10, 47.4) centre (10.5, 47.4) ccw projected
  line L3 (10, 47.4) -> (10, 36.65) projected
  arc A308 (9.5, 36.15) -> (10, 36.65) centre (9.5, 36.65) ccw projected
  line L4 (9.5, 36.15) -> (0.5, 36.15) projected
  line L5 (0, 35.65) -> (0.5, 36.15) projected
  line L6 (0, 35.65) -> (0, 25.45) projected
  line L7 (0.5, 24.95) -> (0, 25.45) projected
  line L8 (0.5, 24.95) -> (8.4, 24.95) projected
  arc A309 (8.4, 23.05) -> (8.4, 24.95) centre (8.4, 24) ccw projected
  line L9 (8.4, 23.05) -> (0.5, 23.05) projected
  line L10 (0, 22.55) -> (0.5, 23.05) projected
  line L11 (0, 22.55) -> (0, -14.65) projected
  line L12 (0.5, -15.15) -> (0, -14.65) projected
  line L13 (0.5, -15.15) -> (10, -15.15) projected
  arc A310 (10, -18.65) -> (10, -15.15) centre (10, -16.9) ccw projected
  line L14 (10, -18.65) -> (2.5, -18.65) projected
  arc A311 (2.5, -18.65) -> (2, -19.15) centre (2.5, -19.15) ccw projected
  line L15 (2, -19.15) -> (2, -47.4) projected
  arc A312 (2, -47.4) -> (2.5, -47.9) centre (2.5, -47.4) ccw projected
  line L16 (2.5, -47.9) -> (89.9, -47.9) projected
  arc A313 (89.9, -47.9) -> (90.4, -47.4) centre (89.9, -47.4) ccw projected
  line L17 (90.4, -47.4) -> (90.4, -5) projected
  arc A314 (36.05, -1.5) -> (34.05, -3.5) centre (36.05, -3.5) ccw projected
  line L18 (36.05, -1.5) -> (49.05, -1.5) projected
  arc A315 (51.05, -3.5) -> (49.05, -1.5) centre (49.05, -3.5) ccw projected
  line L19 (51.05, -3.5) -> (51.05, -24.5) projected
  arc A316 (49.05, -26.5) -> (51.05, -24.5) centre (49.05, -24.5) ccw projected
  line L20 (49.05, -26.5) -> (36.05, -26.5) projected
  arc A317 (34.05, -24.5) -> (36.05, -26.5) centre (36.05, -24.5) ccw projected
  line L21 (34.05, -24.5) -> (34.05, -3.5) projected
  arc A318 (36.05, 26.5) -> (34.05, 24.5) centre (36.05, 24.5) ccw projected
  line L22 (36.05, 26.5) -> (49.05, 26.5) projected
  arc A319 (51.05, 24.5) -> (49.05, 26.5) centre (49.05, 24.5) ccw projected
  line L23 (51.05, 24.5) -> (51.05, 3.5) projected
  arc A320 (49.05, 1.5) -> (51.05, 3.5) centre (49.05, 3.5) ccw projected
  line L24 (49.05, 1.5) -> (36.05, 1.5) projected
  arc A321 (34.05, 3.5) -> (36.05, 1.5) centre (36.05, 3.5) ccw projected
  line L25 (34.05, 3.5) -> (34.05, 24.5) projected
  point P0 (0, 0)
  point P1 (1.5, -44.9)
  point P2 (1.5, -43.9)
  point P3 (1.5, -42.9)
  point P4 (1.5, -41.9)
  point P5 (1.5, -40.9)
  point P6 (1.5, -39.9)
  point P7 (1.5, -38.9)
  point P8 (1.5, -37.9)
  point P9 (1.5, -36.9)
  point P10 (1.5, -35.9)
  point P11 (1.5, -34.9)
  point P12 (1.5, -33.9)
  point P13 (1.5, -32.9)
  point P14 (1.5, -31.9)
  point P15 (1.5, -30.9)
  point P16 (1.5, -29.9)
  point P17 (1.5, -28.9)
  point P18 (1.5, -27.9)
  point P19 (1.5, -26.9)
  point P20 (1.5, -25.9)
  point P21 (1.5, -24.9)
  point P22 (1.5, -23.9)
  point P23 (1.5, -22.9)
  point P24 (1.5, -21.9)
  point P25 (1.5, -20.9)
  point P26 (0.5, -44.9)
  point P27 (0.5, -43.9)
  point P28 (0.5, -42.9)
  point P29 (0.5, -41.9)
  point P30 (0.5, -40.9)
  point P31 (0.5, -39.9)
  point P32 (0.5, -38.9)
  point P33 (0.5, -37.9)
  point P34 (0.5, -36.9)
  point P35 (0.5, -35.9)
  point P36 (0.5, -34.9)
  point P37 (0.5, -33.9)
  point P38 (0.5, -32.9)
  point P39 (0.5, -31.9)
  point P40 (0.5, -30.9)
  point P41 (0.5, -29.9)
  point P42 (0.5, -28.9)
  point P43 (0.5, -27.9)
  point P44 (0.5, -26.9)
  point P45 (0.5, -25.9)
  point P46 (0.5, -24.9)
  point P47 (0.5, -23.9)
  point P48 (0.5, -22.9)
  point P49 (0.5, -21.9)
  point P50 (0.5, -20.9)
  dimension "d205" = 0.5
  dimension "d206" = 3
  dimension "d209" = 1
  dimension "d212" = 1
  constraints: 1 horizontal, 1 vertical, 49 other
  measures "d205" distance from line of point (1.5, -44.9) L15
  measures "d206" distance from line of L16 point (1.5, -44.9)
  measures "d209" distance of point (1.5, -44.9) point (1.5, -43.9)
  measures "d212" distance of point (1.5, -44.9) point (0.5, -44.9)
equation "\"d23\" = d22"
equation "\"d25\" = d22"
equation "\"d42\" = d39"
equation "\"d45\" = d39"
body "Solid1"
